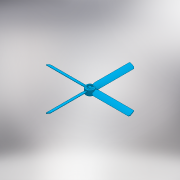
# Autodesk Inventor part: 40x40x4 CW Prop Blue
Saved by Autodesk Inventor 2018 (Build 220112000, 112)
## iProperties
Created: 2018-01-07
Part Number: 40x40x4 CW Prop Blue
Material: Nylon 6/6
Document SubType Name: Modeling
Designer: fbl92568
Density: 1.13 g/cm^3
Appearance: Sky Blue Medium
Author: fbl92568
Autodesk Inventor part; units mm, degrees
ref_plane "YZ Plane" through (0, 0, 0) normal (1, 0, 0) x (0, 1, 0)
ref_plane "XZ Plane" through (0, 0, 0) normal (0, 1, 0) x (-1, 0, 0)
ref_plane "XY Plane" through (0, 0, 0) normal (0, 0, 1) x (1, 0, 0)
sketch "Sketch1" plane through (0, 0, 0) normal (0, 0, 1) x (1, 0, 0)
  circle A0 centre (0, 0) radius 2.5
  circle A1 centre (0, 0) radius 5
  dimension "d0" = 5
  dimension "d1" = 10
  constraints: 2 centre point, 2 coincident
  measures "d0" diameter of A0
  measures "d1" diameter of A1
extrude "Extrusion1" add sketch "Sketch1" along normal blind 7
sketch "Sketch2" plane through (0, 0, 7) normal (0, 0, 1) x (1, 0, 0)
  circle A0 centre (0, 0) radius 3
  dimension "d4" = 6
  constraints: 1 centre point, 1 coincident
  measures "d4" diameter of A0
extrude "Extrusion2" cut sketch "Sketch2" against normal blind 3
fillet "Fillet1" radius 1 2 edges at (-5, 0, 7) (-5, 0, 0)
sketch "Sketch3" plane through (0, 0, 0) normal (1, 0, 0) x (0, 1, 0)
  line L0 (2.5312, 5.9831) -> (-0.7595, 4.8545) construction
  line L1 (-0.7595, 4.8545) -> (-3.373, 2.7518) construction
  spline S0 degree 2 poles (2.5312, 5.9831) (-0.7595, 4.8545) (-3.373, 2.7518) knots 1 1 1 2 2 2
  line L2 (2.5264, 5.5288) -> (-0.3988, 3.8033) construction
  line L3 (-0.3988, 3.8033) -> (-3.182, 2.5147) construction
  spline S1 degree 2 poles (2.5264, 5.5288) (-0.3988, 3.8033) (-3.182, 2.5147) knots 1 1 1 2 2 2
  arc A0 (2.5264, 5.5288) -> (2.5312, 5.9831) centre (2.3916, 5.7574) ccw
  arc A1 (-3.373, 2.7518) -> (-3.182, 2.5147) centre (-3.2665, 2.6421) ccw
  point P0 (0, 0)
  constraints: 4 point on circle, 2 centre point, 1 tangent, 6 other
extrude "Extrusion3" add sketch "Sketch3" along normal blind 50
sketch "Sketch4" plane through (0, 0, 7) normal (0, 0, 1) x (1, 0, 0)
  circle A0 centre (0, 0) radius 5 projected
  line L0 (4.5163, -2.1454) -> (5.0478, -2.621) construction
  line L1 (5.0478, -2.621) -> (5.618, -3.1462) construction
  line L2 (5.618, -3.1462) -> (7.1686, -3.4205) construction
  spline S0 degree 3 poles (4.5163, -2.1454) (5.0478, -2.621) (5.618, -3.1462) (7.1686, -3.4205) knots 1 1 1 1 2 2 2 2
  line L3 (4.6538, 1.8281) -> (5.3329, 2.2588) construction
  line L4 (5.3329, 2.2588) -> (6.9358, 2.3592) construction
  line L5 (4.2356, 2.657) -> (50, 2.657) projected
  line L6 (6.9358, 2.3592) -> (8.2204, 2.657) construction
  spline S1 degree 3 poles (4.6538, 1.8281) (5.3329, 2.2588) (6.9358, 2.3592) (8.2204, 2.657) knots 1 1 1 1 2 2 2 2
  line L7 (8.2204, 2.657) -> (3.6377, 3.4303)
  line L8 (7.1686, -3.4205) -> (3.3361, -3.7243)
  arc A1 (3.3361, -3.7243) -> (4.5163, -2.1454) centre (0, 0) ccw
  arc A2 (4.6538, 1.8281) -> (3.6377, 3.4303) centre (0, 0) ccw
  constraints: 5 point on circle, 4 end point, 2 centre point, 1 coincident, 1 point on line, 6 other
extrude "Extrusion4" cut sketch "Sketch4" against normal through all contours A0 L5 S1 | S0 L8 A0 | A0 L7 L5
sketch "Sketch5" plane through (0, 0, 7) normal (0, 0, 1) x (1, 0, 0)
  line L0 (7.1626, -3.4194) -> (50, -3.4194) projected
  arc A0 (48.5462, -3.4194) -> (50, -1.9346) centre (46.5228, 0.0157) ccw
  line L1 (8.2204, 2.657) -> (50, 2.657) projected
  arc A1 (50, 1.6991) -> (48.9788, 2.657) centre (48.9528, 1.6059) ccw
  line L2 (48.9788, 2.657) -> (49.1315, 2.7527)
  line L3 (49.1315, 2.7527) -> (50.2481, 2.7048)
  line L4 (50.2481, 2.7048) -> (50, 1.6991)
  line L5 (48.5462, -3.4194) -> (50.0712, -3.5566)
  line L6 (50.0712, -3.5566) -> (50, -1.9346)
  point P0 (0, 0)
  constraints: 10 end point, 4 point on circle, 2 centre point, 2 point on line
extrude "Extrusion5" cut sketch "Sketch5" against normal through all
pattern_circular "Circular Pattern1" count 4 over 360 about axis through (0, 0, -10) along (0, 0, 1) of "Extrusion3", "Extrusion4", "Extrusion5"
body "Solid1"
